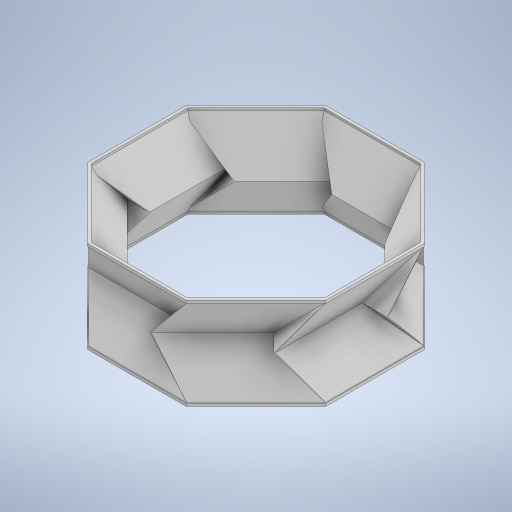
# Autodesk Inventor part: 팔각형 OV-PAM 층 한개
Saved by Autodesk Inventor 2024 (Build 280153000, 153)
## iProperties
Created: 2023-06-16
Part Number: 팔각형 OV-PAM 층 한개
Material: 일반
Document SubType Name: Modeling
Designer: jsw
Density: 1 g/cm^3
Appearance: 기본값
Author: jsw
Autodesk Inventor part; units mm, degrees
ref_plane "YZ Plane" through (0, 0, 0) normal (1, 0, 0) x (0, 1, 0)
ref_plane "XZ Plane" through (0, 0, 0) normal (0, 1, 0) x (-1, 0, 0)
ref_plane "XY Plane" through (0, 0, 0) normal (0, 0, 1) x (1, 0, 0)
sketch "스케치1" plane through (0, 0, 0) normal (0, 1, 0) x (-1, 0, 0)
  line L0 (-32.5919, 13.5) -> (-13.5, 32.5919)
  line L1 (-13.5, 32.5919) -> (13.5, 32.5919)
  line L2 (13.5, 32.5919) -> (32.5919, 13.5)
  line L3 (32.5919, 13.5) -> (32.5919, -13.5)
  line L4 (32.5919, -13.5) -> (13.5, -32.5919)
  line L5 (13.5, -32.5919) -> (-13.5, -32.5919)
  line L6 (-13.5, -32.5919) -> (-32.5919, -13.5)
  line L7 (-32.5919, -13.5) -> (-32.5919, 13.5)
  line L8 (-13.6657, 32.9919) -> (13.6657, 32.9919)
  line L9 (13.6657, 32.9919) -> (32.9919, 13.6657)
  line L10 (32.9919, 13.6657) -> (32.9919, -13.6657)
  line L11 (32.9919, -13.6657) -> (13.6657, -32.9919)
  line L12 (13.6657, -32.9919) -> (-13.6657, -32.9919)
  line L13 (-13.6657, -32.9919) -> (-32.9919, -13.6657)
  line L14 (-32.9919, -13.6657) -> (-32.9919, 13.6657)
  line L15 (-32.9919, 13.6657) -> (-13.6657, 32.9919)
  point P0 (0, 0)
  point P1 (0, 0)
  point P2 (0, 0)
  dimension "d0" = 27
  dimension "d2" = 0.4
  constraints: 32 end point, 2 coincident, 2 horizontal, 34 other
  measures "d0" distance of L0.end L1.end
  measures "d2" distance between parallel lines of L10 L3
extrude "돌출2" add sketch "스케치1" along normal blind 12 contours L0 L1 L2 L3 L4 L5 L6 L7 | L8 L9 L10 L11 L12 L13 L14 L15
ref_plane "작업 평면2" through (32.9919, 0, 13.6657) normal (-0.8660254, -0.5, 0) x (0, 0, -1)
sketch "스케치3" plane through (32.9919, 0, 13.6657) normal (1, 0, 0) x (0, 0, -1)
  line L0 (0, 0) -> (0, 12) projected
  line L1 (0, 12) -> (27.3314, 12) projected
  line L2 (0, 0) -> (27.3314, 0)
  line L3 (27.3314, 0) -> (27.3314, 12)
  line L4 (27.3314, 12) -> (0, 12)
  line L5 (0, 12) -> (0, 0)
  line L6 (0, 12) -> (-7.3047, 12)
  line L7 (-19.3262, 12) -> (0, 12) projected
  line L8 (0, 0) -> (-7.3047, 12)
  line L9 (27.3314, 12) -> (13.6657, 12)
  line L10 (17.1657, 12) -> (27.3314, 0)
  point P0 (13.6657, 0)
  point P1 (17.1657, 12)
  dimension "d17" = 121.33
  dimension "d49" = 3.5
  constraints: 16 end point, 5 midpoint, 2 parallel, 2 point on line, 1 horizontal, 1 perpendicular
  measures "d17" angle of L8 L2
  measures "d49" distance of point (13.666, 12) L10.start
extrude "돌출4" cut sketch "스케치3" against normal up to surface contours L8 L6 L0 | L0 L1 L10 L2 surface through (32.9919, 0, 13.6657) normal (-0.8660254, -0.5, 0)
pattern_circular "원형 패턴1" count 8 over 360 about axis through (0, -10, 0) along (0, 1, 0) of "돌출4"
mirror "미러5" about plane through (0, 12, 0) normal (0, 1, 0) of "돌출2", "돌출4", "원형 패턴1"
sketch "스케치9" plane through (-13.6657, 24, -32.9919) normal (0, 1, 0) x (1, 0, 0)
  line L0 (46.6576, -46.6576) -> (46.6576, -19.3262) projected
  line L1 (46.6576, -19.3262) -> (27.3314, 0) projected
  line L2 (27.3314, 0) -> (0, 0) projected
  line L3 (0, 0) -> (-19.3262, -19.3262) projected
  line L4 (-19.3262, -19.3262) -> (-19.3262, -46.6576) projected
  line L5 (-19.3262, -46.6576) -> (0, -65.9838) projected
  line L6 (0, -65.9838) -> (27.3314, -65.9838) projected
  line L7 (27.3314, -65.9838) -> (46.6576, -46.6576) projected
  point P0 (13.6657, -32.9919)
extrude "돌출8" add sketch "스케치9" along normal blind 0.8
sketch "스케치10" plane through (0, 0, 0) normal (0, -1, 0) x (1, 0, 0)
  line L0 (32.9919, 13.6657) -> (32.9919, -13.6657) projected
  line L1 (13.6657, 32.9919) -> (32.9919, 13.6657) projected
  line L2 (-13.6657, 32.9919) -> (13.6657, 32.9919) projected
  line L3 (-32.9919, 13.6657) -> (-13.6657, 32.9919) projected
  line L4 (-32.9919, -13.6657) -> (-32.9919, 13.6657) projected
  line L5 (-13.6657, -32.9919) -> (-32.9919, -13.6657) projected
  line L6 (13.6657, -32.9919) -> (-13.6657, -32.9919) projected
  line L7 (32.9919, -13.6657) -> (13.6657, -32.9919) projected
  point P0 (0, 0)
extrude "돌출9" add sketch "스케치10" along normal blind 0.8
shell "쉘6" thickness 0.6 removed faces 2 at (4.5552, 24.8, 10.9973) at (4.5552, -0.8, 10.9973)
sketch "스케치12" plane through (-13.6657, 24.8, -32.9919) normal (0, 1, 0) x (1, 0, 0)
  line L0 (46.0576, -19.5747) -> (46.0576, -46.409) projected
  line L1 (46.0576, -46.409) -> (27.0828, -65.3838) projected
  line L2 (27.0828, -65.3838) -> (0.2485, -65.3838) projected
  line L3 (0.2485, -65.3838) -> (-18.7262, -46.409) projected
  line L4 (-18.7262, -46.409) -> (-18.7262, -19.5747) projected
  line L5 (-18.7262, -19.5747) -> (0.2485, -0.6) projected
  line L6 (0.2485, -0.6) -> (27.0828, -0.6) projected
  line L7 (27.0828, -0.6) -> (46.0576, -19.5747) projected
  line L8 (46.6576, -19.3262) -> (27.3314, 0) projected
  line L9 (27.3314, 0) -> (0, 0) projected
  line L10 (0, 0) -> (-19.3262, -19.3262) projected
  line L11 (-19.3262, -19.3262) -> (-19.3262, -46.6576) projected
  line L12 (-19.3262, -46.6576) -> (0, -65.9838) projected
  line L13 (0, -65.9838) -> (27.3314, -65.9838) projected
  line L14 (27.3314, -65.9838) -> (46.6576, -46.6576) projected
  line L15 (46.6576, -46.6576) -> (46.6576, -19.3262) projected
  line L16 (-0.0828, 0.2) -> (27.4142, 0.2)
  line L17 (27.4142, 0.2) -> (46.8576, -19.2434)
  line L18 (46.8576, -19.2434) -> (46.8576, -46.7404)
  line L19 (46.8576, -46.7404) -> (27.4142, -66.1838)
  line L20 (27.4142, -66.1838) -> (-0.0828, -66.1838)
  line L21 (-0.0828, -66.1838) -> (-19.5262, -46.7404)
  line L22 (-19.5262, -46.7404) -> (-19.5262, -19.2434)
  line L23 (-19.5262, -19.2434) -> (-0.0828, 0.2)
  point P0 (13.6657, -32.9919)
  point P1 (13.6657, -32.9919)
  dimension "d50" = 0.2
  constraints: 16 end point, 1 coincident, 1 horizontal, 17 other
  measures "d50" distance between parallel lines of L9 L16
extrude "돌출10" add sketch "스케치12" against normal blind 0.8 contours L16 L17 L18 L19 L20 L21 L22 L23
ref_plane "작업 평면6" through (-13.6657, 12, -32.9919) normal (0, 1, 0) x (1, 0, 0)
mirror "미러8" about plane through (-13.6657, 12, -32.9919) normal (0, 1, 0) of "돌출10"
